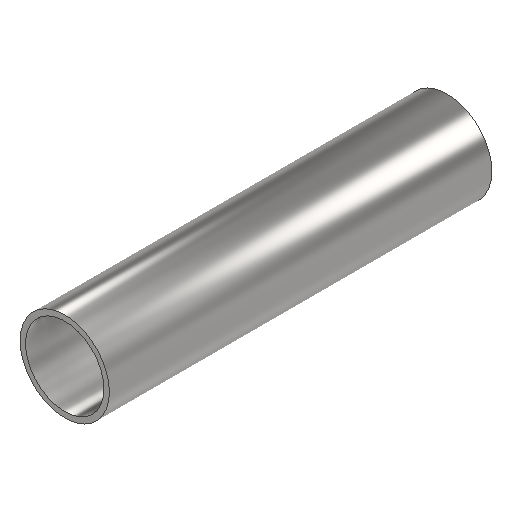
# Autodesk Inventor part: ICF34_70mmNipplePipe
Saved by Autodesk Inventor 2026.2 (Build 302298000, 298)
## iProperties
Created: 2023-07-13
Part Number: ICF34_70mmNipplePipe
Material: ステンレス鋼 440C
Document SubType Name: Modeling
Designer: kuzmin
Density: 7.75 g/cm^3
Appearance: 半つや出し
Author: kuzmin
Autodesk Inventor part; units mm, degrees
ref_plane "YZ Plane" through (0, 0, 0) normal (1, 0, 0) x (0, 1, 0)
ref_plane "XZ Plane" through (0, 0, 0) normal (0, 1, 0) x (-1, 0, 0)
ref_plane "XY Plane" through (0, 0, 0) normal (0, 0, 1) x (1, 0, 0)
sketch "Sketch1" plane through (0, 0, 0) normal (0, 0, 1) x (1, 0, 0)
  circle A0 centre (0, 0) radius 7.17
  circle A1 centre (0, 0) radius 8.17
  dimension "d0" = 16.34
  dimension "d1" = 1
  constraints: 2 centre point, 2 coincident
  measures "d0" diameter of A1
  measures "d1" radial gap between concentric circles of A0 A1
extrude "Extrusion1" add sketch "Sketch1" along normal blind 70
body "Solid1"
